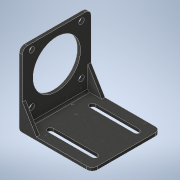
# Autodesk Inventor part: NEMA23_StepperonlineMount
Saved by Autodesk Inventor 2021 (Build 250183000, 183)
## iProperties
Created: 2021-01-25
Part Number: NEMA23_StepperonlineMount
Material: Generic
Document SubType Name: Modeling
Designer: Jorian Brusind
Density: 1 g/cm^3
Appearance: Fine Textured - Black
Mass: 21.0234 g
Surface Area: 162.552 cm^2
Volume: 21.0234 cm^3
Author: Jorian Brusind
Autodesk Inventor part; units mm, degrees
ref_plane "YZ Plane" through (0, 0, 0) normal (1, 0, 0) x (0, 1, 0)
ref_plane "XZ Plane" through (0, 0, 0) normal (0, 1, 0) x (-1, 0, 0)
ref_plane "XY Plane" through (0, 0, 0) normal (0, 0, 1) x (1, 0, 0)
sketch "Sketch1" plane through (0, 0, 0) normal (0, 1, 0) x (-1, 0, 0)
  line L0 (0, 0) -> (69, 0)
  line L1 (69, 0) -> (69, -65)
  line L2 (69, -65) -> (0, -65)
  line L3 (0, -65) -> (0, 0)
  dimension "d0" = 69
  dimension "d1" = 65
  constraints: 8 end point, 2 parallel, 1 horizontal, 1 perpendicular
  measures "d0" distance of L1.end L2.end
  measures "d1" distance of L0.end L1.end
extrude "Extrusion1" add sketch "Sketch1" along normal blind 3
sketch "Sketch2" plane through (0, 3, 0) normal (0, 1, 0) x (1, 0, 0)
  line L0 (0, 65) -> (-69, 65) projected
  line L1 (-69, 65) -> (-66, 65)
  line L2 (-66, 65) -> (-66, 0)
  line L3 (-66, 0) -> (-69, 0)
  line L4 (-69, 0) -> (-69, 65)
  point P0 (0, 0)
  dimension "d4" = 3
  dimension "d5" = 65
  constraints: 8 end point, 2 parallel, 1 horizontal, 1 perpendicular
  measures "d4" distance of L2.end L3.end
  measures "d5" distance of L1.end L2.end
extrude "Extrusion2" add sketch "Sketch2" along normal blind 66
fillet "Fillet1" radius 2 2 edges at (-66, 3, -32.5) (-69, 0, -32.5)
sketch "Sketch3" plane through (0, 0, 0) normal (0, 0, 1) x (1, 0, 0)
  line L0 (-67, 0) -> (0, 0) projected
  line L1 (-66, 0) -> (-51, 0) construction
  line L2 (-66, 5) -> (-66, 69) projected
  line L3 (-66, 5) -> (-66, 0)
  line L4 (-66, 5) -> (-61, 5) construction
  line L5 (-66, 0) -> (-51, 0)
  line L6 (-66, 0) -> (-66, 25)
  line L7 (-66, 25) -> (-51, 0)
  dimension "d12" = 5
  dimension "d13" = 90
  dimension "d14" = 15
  dimension "d15" = 90
  dimension "d16" = 25
  constraints: 12 end point, 3 perpendicular, 2 horizontal, 1 point on line
  measures "d12" distance of L2.start L1.start
  measures "d13" angle of L3 L4
  measures "d14" distance of L1.start L1.end
  measures "d15" angle of L5 L3
  measures "d16" distance of L1.start L6.end
extrude "Extrusion3" add sketch "Sketch3" against normal blind 3
pattern_linear "Rectangular Pattern1" count 2 spacing 62 along (0, 0, -1) of "Extrusion3"
sketch "Sketch4" plane through (-66, 69, 0) normal (1, 0, 0) x (0, 0, -1)
  circle A0 centre (32.5, -29) radius 22.5
  line L0 (0, 0) -> (65, 0) projected
  line L1 (0, -44) -> (0, 0) projected
  point P0 (0, -69)
  dimension "d22" = 45
  dimension "d23" = 29
  dimension "d24" = 32.5
  constraints: 1 centre point
  measures "d22" diameter of A0
  measures "d23" distance from line of L0 A0.centre
  measures "d24" distance from line of L1 A0.centre
extrude "Extrusion4" cut sketch "Sketch4" against normal blind 3
sketch "Sketch5" plane through (-66, 69, 0) normal (1, 0, 0) x (0, 0, -1)
  circle A0 centre (9, -5.501) radius 2.6
  line L0 (0, 0) -> (65, 0) projected
  line L1 (0, -44) -> (0, 0) projected
  circle A1 centre (56, -5.501) radius 2.6
  circle A2 centre (9, -52.501) radius 2.6
  circle A3 centre (56, -52.501) radius 2.6
  point P0 (0, -69)
  dimension "d27" = 5.2
  dimension "d28" = 5.501
  dimension "d29" = 9
  dimension "d32" = 47
  dimension "d35" = 47
  constraints: 4 centre point, 1 horizontal, 1 vertical, 6 other
  measures "d27" diameter of A0
  measures "d28" distance from line of L0 A0.centre
  measures "d29" distance from line of L1 A0.centre
  measures "d32" distance of A0.centre A1.centre
  measures "d35" distance of A0.centre A2.centre
extrude "Extrusion5" cut sketch "Sketch5" against normal blind 3
sketch "Sketch6" plane through (0, 3, 0) normal (0, 1, 0) x (1, 0, 0)
  line L0 (-52.8, 0) -> (0, 0) projected
  line L1 (0, 0) -> (0, 65) projected
  arc A0 (-51.9673, 15.2498) -> (-52, 9.75) centre (-52, 12.5) ccw
  line L2 (-69, 65) -> (-69, 0) projected
  line L3 (-11.5517, 12.5) -> (-9.4517, 12.5) construction
  line L4 (-11.5517, 9.75) -> (-52, 9.75)
  line L5 (-52, 12.5) -> (-10, 12.5) construction
  line L6 (-52, 9.75) -> (-10, 9.75)
  line L7 (-10, 15.25) -> (-52, 15.25)
  arc A1 (-52, 15.25) -> (-52, 9.75) centre (-52, 12.5) ccw
  arc A2 (-10, 9.75) -> (-10, 15.25) centre (-10, 12.5) ccw
  point P0 (-31, 12.5)
  dimension "d48" = 5.5
  dimension "d49" = 12.5
  dimension "d50" = 12.5
  dimension "d54" = 17
  dimension "d62" = 42
  dimension "d63" = 5.5
  constraints: 12 end point, 6 point on circle, 4 tangent, 3 centre point, 1 horizontal, 1 midpoint, 1 parallel, 1 point on line
  measures "d48" diameter of A0
  measures "d49" distance from line of L0 L3.start
  measures "d50" distance from line of L0 L5.start
  measures "d54" distance from line of L2 L5.start
  measures "d62" distance of L5.start L5.end
  measures "d63" diameter of A2
extrude "Extrusion6" cut sketch "Sketch6" against normal blind 3
pattern_linear "Rectangular Pattern2" count 2 spacing 40 along (0, 0, -1) of "Extrusion6"
fillet "Fillet2" radius 5 2 edges at (-67.5, 69, 0) (-67.5, 69, -65)
fillet "Fillet3" radius 5 2 edges at (0, 1.5, 0) (0, 1.5, -65)
body "Solid1"
